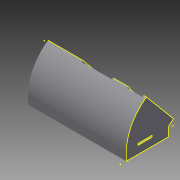
# Autodesk Inventor part: rrd display
Saved by Autodesk Inventor 2014 (Build 180170000, 170)
## iProperties
Created: 2013-09-12
Part Number: rrd display
Material: Generic
Document SubType Name: Modeling
Designer: stephen
Density: 1 g/cm^3
Appearance: Default
Author: stephen
Autodesk Inventor part; units mm, degrees
ref_plane "YZ Plane" through (0, 0, 0) normal (1, 0, 0) x (0, 1, 0)
ref_plane "XZ Plane" through (0, 0, 0) normal (0, 1, 0) x (-1, 0, 0)
ref_plane "XY Plane" through (0, 0, 0) normal (0, 0, 1) x (1, 0, 0)
sketch "Sketch1" plane through (0, 0, 0) normal (0, 0, 1) x (1, 0, 0)
  line L0 (203.8319, 85.6077) -> (27.8319, 85.6077)
  line L1 (27.8319, 85.6077) -> (27.8319, 10.1077)
  line L2 (27.8319, 10.1077) -> (203.8319, 10.1077)
  line L3 (203.8319, 10.1077) -> (203.8319, 85.6077)
  line L4 (88.1319, 64.3077) -> (185.5319, 64.3077)
  line L5 (185.5319, 64.3077) -> (185.5319, 23.9077)
  line L6 (185.5319, 23.9077) -> (88.1319, 23.9077)
  line L7 (88.1319, 23.9077) -> (88.1319, 64.3077)
  circle A0 centre (63.3719, 47.7577) radius 3.5
  circle A1 centre (63.3719, 67.0777) radius 1
  circle A2 centre (59.5619, 67.0777) radius 1
  circle A3 centre (67.1819, 67.0777) radius 1
  line L8 (65.9589, 30.9177) -> (60.7989, 30.9177) construction
  line L9 (65.9589, 33.8177) -> (60.7989, 33.8177)
  line L10 (60.7989, 28.0177) -> (65.9589, 28.0177)
  arc A4 (65.9589, 28.0177) -> (65.9589, 33.8177) centre (65.9589, 30.9177) ccw
  arc A5 (60.7989, 33.8177) -> (60.7989, 28.0177) centre (60.7989, 30.9177) ccw
  line L11 (60.7989, 30.9177) -> (65.9589, 30.9177) construction
  line L12 (60.7989, 36.3177) -> (65.9589, 36.3177)
  line L13 (65.9589, 25.5177) -> (60.7989, 25.5177)
  circle A6 centre (55.7989, 30.9177) radius 0.8
  arc A7 (55.7989, 33.8477) -> (55.7989, 27.9877) centre (55.7989, 30.9177) ccw
  line L14 (52.8689, 30.9177) -> (52.156, 30.9177)
  circle A8 centre (70.9589, 30.9177) radius 0.8
  arc A9 (70.9589, 27.9877) -> (70.9589, 33.8477) centre (70.9589, 30.9177) ccw
  line L15 (55.7989, 33.8477) -> (56.263, 33.8477)
  line L16 (55.7989, 27.9877) -> (56.263, 27.9877)
  line L17 (70.9589, 33.8477) -> (70.4949, 33.8477)
  line L18 (70.9589, 27.9877) -> (70.4949, 27.9877)
  arc A10 (65.9589, 25.5177) -> (70.4949, 27.9877) centre (65.9589, 30.9177) ccw
  arc A11 (70.4949, 33.8477) -> (65.9589, 36.3177) centre (65.9589, 30.9177) ccw
  line L19 (63.3789, 30.9177) -> (63.6989, 30.9177)
  arc A12 (60.7989, 36.3177) -> (56.263, 33.8477) centre (60.7989, 30.9177) ccw
  arc A13 (56.263, 27.9877) -> (60.7989, 25.5177) centre (60.7989, 30.9177) ccw
  line L20 (49.2039, 75.3911) -> (49.2038, 75.3911)
  line L21 (197.3319, 23.9109) -> (197.3319, 23.9077)
  line L22 (34.8319, 58.2326) -> (47.1919, 58.2326)
  line L23 (47.1919, 58.2326) -> (47.1919, 37.3026)
  line L24 (47.1919, 37.3026) -> (34.8319, 37.3026)
  line L25 (34.8319, 37.3026) -> (34.8319, 58.2326)
  line L26 (63.3719, 47.7577) -> (63.3818, 51.2577)
  line L27 (63.3719, 47.7577) -> (59.872, 47.7675)
  circle A14 centre (52.0039, 25.4109) radius 1.5
  circle A15 centre (52.0039, 75.4645) radius 1.5
  circle A16 centre (197.004, 75.4645) radius 1.5
  circle A17 centre (197.3319, 25.4109) radius 1.5
  line L28 (63.3789, 36.3177) -> (63.386, 38.8177)
  point P0 (0, 0)
  dimension "d53" = 3
  dimension "d0" = 176
  dimension "d1" = 75.5
  dimension "d2" = 97.4
  dimension "d3" = 40.4
  dimension "d4" = 13.8
  dimension "d5" = 18.3
  dimension "d6" = 21.26
  dimension "d7" = 7
  dimension "d8" = 34.15
  dimension "d9" = 10.96
  dimension "d10" = 5.8
  dimension "d11" = 0.007
  dimension "d12" = 7.94
  dimension "d16" = 1.6
  dimension "d17" = 10.8
  dimension "d19" = 2.13
  dimension "d20" = 0
  dimension "d21" = 1.6
  dimension "d22" = 2.13
  dimension "d24" = 2
  dimension "d25" = 1.81
  dimension "d26" = 1.81
  dimension "d27" = 0
  dimension "d28" = 14.82
  dimension "d36" = 0
  dimension "d43" = 5
  dimension "d44" = 5
  dimension "d45" = 12.36
  dimension "d46" = 20.93
  dimension "d47" = 7
  dimension "d50" = 3
  dimension "d51" = 3
  dimension "d52" = 3
  dimension "d55" = 10.1432
  dimension "d56" = 10.1432
  dimension "d57" = 15.3032
  dimension "d58" = 15.3032
  dimension "d184" = 2.5
  constraints: 62 end point, 20 point on circle, 17 centre point, 15 parallel, 12 tangent, 6 coincident, 6 perpendicular, 3 horizontal, 3 midpoint, 2 collinear, 2 equal radius, 2 point on line, 1 vertical alignment, 2 other
  measures "d0" distance of L0.start L0.end
  measures "d1" distance of L0.end L1.end
  measures "d2" distance of L4.start L4.end
  measures "d3" distance of L6.end L4.start
  measures "d4" distance between parallel lines of L2 L6
  measures "d5" distance between parallel lines of L3 L5
  measures "d6" distance edge to line of A0 L7
  measures "d7" diameter of A0
  measures "d8" distance edge to line of A0 L2
  measures "d10" distance between parallel lines of L9 L10
  measures "d11" horizontal distance of point (63.379, 30.918) L26.start
  measures "d12" distance edge to line of A0 L12
  measures "d16" diameter of A6
  measures "d17" distance between parallel lines of L12 L13
  measures "d19" radial gap between concentric circles of A7 A6
  measures "d20" distance from line of L14 A6.centre
  measures "d21" diameter of A8
  measures "d22" radial gap between concentric circles of A9 A8
  measures "d24" diameter of A1
  measures "d27" horizontal distance of L26.start A1.centre
  measures "d36" horizontal distance of point (52.004, 25.411) point (52.004, 75.465)
  measures "d43" distance of L8.start A8.centre
  measures "d44" distance of L8.end A6.centre
  measures "d45" distance of L22.end L22.start
  measures "d46" distance of L24.end L22.start
  measures "d47" distance from line of L1 L22.start
  measures "d50" diameter of A14
  measures "d51" diameter of A15
  measures "d52" diameter of A16
  measures "d55" distance from line of L0 point (52.004, 75.465)
  measures "d56" distance from line of L0 A16.centre
  measures "d57" distance from line of L2 point (197.332, 25.411)
  measures "d58" distance from line of L2 point (52.004, 25.411)
  measures "d184" distance of L28.start L28.end
extrude "Extrusion3" add sketch "Sketch1" along normal blind 2 contours L3 L2 L1 L0
sketch "Sketch3" plane through (0, 0, 2) normal (0, 0, 1) x (1, 0, 0)
  line L0 (203.8319, 85.6077) -> (27.8319, 85.6077) projected
  line L1 (27.8319, 85.6077) -> (27.8319, 10.1077) projected
  line L2 (27.8319, 10.1077) -> (203.8319, 10.1077) projected
  line L3 (203.8319, 10.1077) -> (203.8319, 85.6077) projected
  line L4 (30.8319, 82.6077) -> (200.8319, 82.6077)
  line L5 (200.8319, 82.6077) -> (200.8319, 13.1077)
  line L6 (200.8319, 13.1077) -> (30.8319, 13.1077)
  line L7 (30.8319, 13.1077) -> (30.8319, 82.6077)
  point P0 (0, 0)
  dimension "d63" = 3
  dimension "d64" = 3
  dimension "d65" = 3
  dimension "d66" = 3
  constraints: 8 end point, 2 parallel, 1 horizontal, 1 perpendicular
  measures "d63" distance between parallel lines of L0 L4
  measures "d64" distance between parallel lines of L2 L6
  measures "d65" distance between parallel lines of L1 L7
  measures "d66" distance between parallel lines of L3 L5
extrude "Extrusion4" add sketch "Sketch3" along normal blind 14
sketch "Sketch4" plane through (0, 0, 2) normal (0, 0, 1) x (1, 0, 0)
  circle A0 centre (52.0039, 25.4109) radius 1.5 projected
  circle A1 centre (52.0039, 75.4645) radius 1.5 projected
  circle A2 centre (197.004, 75.4645) radius 1.5 projected
  circle A3 centre (197.3319, 25.4109) radius 1.5 projected
  circle A4 centre (52.0039, 75.4645) radius 2.5
  circle A5 centre (197.004, 75.4645) radius 2.5
  circle A6 centre (197.3319, 25.4109) radius 2.5
  circle A7 centre (52.0039, 25.4109) radius 2.5
  point P0 (0, 0)
  dimension "d69" = 5
  dimension "d70" = 5
  dimension "d71" = 5
  dimension "d72" = 5
  constraints: 4 centre point, 4 coincident
  measures "d69" diameter of A4
  measures "d70" diameter of A5
  measures "d71" diameter of A6
  measures "d72" diameter of A7
sketch "Sketch5" plane through (0, 0, 0) normal (0, 0, -1) x (-1, 0, 0)
  arc A0 (-65.9589, 36.3177) -> (-70.4949, 33.8477) centre (-65.9589, 30.9177) ccw projected
  line L0 (-65.9589, 36.3177) -> (-60.7989, 36.3177) projected
  arc A1 (-56.263, 33.8477) -> (-60.7989, 36.3177) centre (-60.7989, 30.9177) ccw projected
  line L1 (-56.263, 33.8477) -> (-55.7989, 33.8477) projected
  arc A2 (-55.7989, 27.9877) -> (-55.7989, 33.8477) centre (-55.7989, 30.9177) ccw projected
  line L2 (-55.7989, 27.9877) -> (-56.263, 27.9877) projected
  arc A3 (-60.7989, 25.5177) -> (-56.263, 27.9877) centre (-60.7989, 30.9177) ccw projected
  line L3 (-60.7989, 25.5177) -> (-65.9589, 25.5177) projected
  arc A4 (-70.4949, 27.9877) -> (-65.9589, 25.5177) centre (-65.9589, 30.9177) ccw projected
  line L4 (-70.4949, 27.9877) -> (-70.9589, 27.9877) projected
  arc A5 (-70.9589, 33.8477) -> (-70.9589, 27.9877) centre (-70.9589, 30.9177) ccw projected
  line L5 (-70.9589, 33.8477) -> (-70.4949, 33.8477) projected
  point P0 (0, 0)
extrude "Extrusion5" add sketch "Sketch5" against normal blind 6.8
sketch "Sketch6" plane through (0, 0, 6.8) normal (0, 0, 1) x (1, 0, 0)
  arc A0 (55.7989, 33.8477) -> (55.7989, 27.9877) centre (55.7989, 30.9177) ccw projected
  arc A1 (70.9589, 27.9877) -> (70.9589, 33.8477) centre (70.9589, 30.9177) ccw projected
  circle A2 centre (55.7989, 30.9177) radius 0.8
  circle A3 centre (70.9589, 30.9177) radius 0.8
  point P0 (0, 0)
  dimension "d75" = 1.6
  dimension "d76" = 1.6
  constraints: 2 centre point, 2 coincident
  measures "d75" diameter of A2
  measures "d76" diameter of A3
extrude "Extrusion6" cut sketch "Sketch6" against normal blind 4.8 contours A3
sketch "Sketch7" plane through (0, 0, 6.8) normal (0, 0, 1) x (1, 0, 0)
  arc A0 (55.7989, 33.8477) -> (55.7989, 27.9877) centre (55.7989, 30.9177) ccw projected
  circle A1 centre (55.7989, 30.9177) radius 0.8
  point P0 (0, 0)
  dimension "d79" = 1.6
  constraints: 1 centre point, 1 coincident
  measures "d79" diameter of A1
extrude "Extrusion7" cut sketch "Sketch7" against normal blind 4.8
sketch "Sketch9" plane through (0, 0, 6.8) normal (0, 0, 1) x (1, 0, 0)
  line L0 (65.9589, 36.3177) -> (60.7989, 36.3177) projected
  arc A0 (56.263, 27.9877) -> (60.7989, 25.5177) centre (60.7989, 30.9177) ccw projected
  arc A1 (65.9589, 25.5177) -> (70.4949, 27.9877) centre (65.9589, 30.9177) ccw projected
  line L1 (65.9589, 30.9177) -> (60.7989, 30.9177) construction
  line L2 (65.9589, 33.8177) -> (60.7989, 33.8177)
  line L3 (60.7989, 28.0177) -> (65.9589, 28.0177)
  arc A2 (65.9589, 28.0177) -> (65.9589, 33.8177) centre (65.9589, 30.9177) ccw
  arc A3 (60.7989, 33.8177) -> (60.7989, 28.0177) centre (60.7989, 30.9177) ccw
  point P0 (0, 0)
  point P1 (63.3789, 30.9177)
  dimension "d83" = 5.8
  constraints: 8 end point, 4 point on circle, 4 tangent, 2 centre point, 2 parallel, 1 midpoint
  measures "d83" diameter of A3
extrude "Extrusion8" cut sketch "Sketch9" against normal blind 6.8
extrude "Extrusion9" add sketch "Sketch4" along normal blind 9.9 contours A7
sketch "Sketch10" plane through (0, 0, 2) normal (0, 0, 1) x (1, 0, 0)
  circle A0 centre (52.0039, 75.4645) radius 1.5 projected
  circle A1 centre (52.0039, 75.4645) radius 2.5
  point P0 (0, 0)
  dimension "d88" = 5
  constraints: 1 centre point, 1 coincident
  measures "d88" diameter of A1
extrude "Extrusion10" add sketch "Sketch10" along normal blind 9.9
sketch "Sketch11" plane through (0, 0, 2) normal (0, 0, 1) x (1, 0, 0)
  circle A0 centre (197.004, 75.4645) radius 1.5 projected
  circle A1 centre (197.004, 75.4645) radius 2.5
  point P0 (0, 0)
  dimension "d91" = 5
  constraints: 1 centre point, 1 coincident
  measures "d91" diameter of A1
extrude "Extrusion11" add sketch "Sketch11" along normal blind 9.9
sketch "Sketch12" plane through (0, 0, 2) normal (0, 0, 1) x (1, 0, 0)
  circle A0 centre (197.3319, 25.4109) radius 1.5 projected
  circle A1 centre (197.3319, 25.4109) radius 2.5
  point P0 (0, 0)
  dimension "d94" = 5
  constraints: 1 centre point, 1 coincident
  measures "d94" diameter of A1
extrude "Extrusion12" add sketch "Sketch12" along normal blind 9.9
sketch "Sketch13" plane through (27.8319, 10.1077, 0) normal (-1, 0, 0) x (0, 0, 1)
  line L0 (16, 75.5) -> (16, 0) projected
  line L1 (16, 75.5) -> (66.453, 33.1649)
  line L2 (16, 75.5) -> (81.8617, 75.5) construction
  line L3 (16, 75.5) -> (23.7135, 84.6925)
  line L4 (23.7135, 84.6925) -> (81.5498, 36.1621)
  line L5 (23.7135, 84.6925) -> (81.5498, 36.1621)
  arc A0 (16, 0) -> (81.5498, 36.1621) centre (12.2266, 84.331) ccw
  point P0 (0, -10.1077)
  dimension "d97" = 40
  dimension "d99" = 12
  dimension "d100" = 75.5
  constraints: 10 end point, 2 point on circle, 1 centre point, 1 equal length, 1 horizontal, 1 perpendicular
  measures "d97" angle of L1 L2
  measures "d99" distance of L0.start L3.end
  measures "d100" distance of L4.end L3.end
extrude "Extrusion13" add sketch "Sketch13" against normal blind 3
sketch "Sketch14" plane through (203.8319, 10.1077, 0) normal (1, 0, 0) x (0, 0, -1)
  line L0 (-16, 0) -> (-16, 75.5) projected
  line L1 (-16, 75.5) -> (-23.7135, 84.6925)
  line L2 (-16, 75.5) -> (-4, 75.5) construction
  line L3 (-23.7135, 84.6925) -> (-81.5498, 36.1621)
  arc A0 (-81.5498, 36.1621) -> (-16, 0) centre (-12.2268, 84.3306) ccw
  point P0 (0, -10.1077)
  dimension "d103" = 12
  dimension "d104" = 130
  dimension "d105" = 75.5
  dimension "d106" = 84.415
  constraints: 6 end point, 2 point on circle, 1 centre point, 1 equal length, 1 horizontal, 1 perpendicular
  measures "d103" distance of L0.end L1.end
  measures "d104" angle of L2 L1
  measures "d105" distance of L1.end L3.end
  measures "d106" radius of A0
extrude "Extrusion14" add sketch "Sketch14" along normal blind 3
sketch "Sketch15" plane through (30.8319, 13.1077, 2) normal (1, 0, 0) x (0, 0, -1)
  line L0 (-14, 72.5) -> (-14, 69.5) projected
  line L1 (-14, 72.5) -> (-21.7135, 81.6925) projected
  line L2 (-21.7135, 81.6925) -> (-79.5498, 33.1621) projected
  arc A0 (-79.5498, 33.1621) -> (-14, -3) centre (-10.2266, 81.331) ccw projected
  line L3 (-14, 0) -> (-14, -3) projected
  line L4 (-14, 69.5) -> (-21.2623, 78.1549)
  line L5 (-21.2623, 78.1549) -> (-75.4966, 32.6469)
  line L6 (-79.5498, 33.1621) -> (-77.2517, 35.0904)
  arc A1 (-75.4966, 32.6469) -> (-14, 0) centre (-10.203, 81.396) ccw
  point P0 (2, -13.1077)
  dimension "d110" = 3
  dimension "d111" = 3
  constraints: 6 end point, 2 perpendicular, 2 point on circle, 1 centre point, 1 point on line
  measures "d110" distance of L2.end L6.end
extrude "Extrusion15" add sketch "Sketch15" along normal blind 173
sketch "Sketch16" plane through (27.8319, 94.8002, 23.7135) normal (0, 0.7660444, 0.6427876) x (1, 0, 0)
  line L0 (179, 0) -> (179, -75.5) projected
  line L1 (0, 0) -> (179, 0) projected
  line L2 (0, -75.5) -> (0, 0) projected
  line L3 (0, -75.5) -> (176, -75.5) projected
  line L4 (3, -3) -> (176, -3)
  line L5 (176, -3) -> (176, -72.5)
  line L6 (176, -72.5) -> (3, -72.5)
  line L7 (3, -72.5) -> (3, -3)
  point P0 (-27.8319, -42.7709)
  dimension "d114" = 3
  dimension "d115" = 3
  dimension "d116" = 3
  dimension "d117" = 3
  constraints: 8 end point, 2 parallel, 1 horizontal, 1 perpendicular
  measures "d114" distance between parallel lines of L2 L7
  measures "d115" distance between parallel lines of L0 L5
  measures "d116" distance between parallel lines of L1 L4
  measures "d117" distance between parallel lines of L3 L6
extrude "Extrusion16" cut sketch "Sketch16" against normal blind 3
sketch "Sketch17" plane through (27.8319, 94.8002, 23.7135) normal (0, 0.7660444, 0.6427876) x (1, 0, 0)
  line L0 (3, -3) -> (176, -3) projected
  line L1 (47.9345, -3) -> (63.9345, -3)
  line L2 (63.9345, -3) -> (63.9345, -13.34)
  line L3 (63.9345, -13.34) -> (47.9345, -13.34)
  line L4 (47.9345, -13.34) -> (47.9345, -3)
  circle A0 centre (55.9345, -8.17) radius 2.55
  circle A1 centre (126.5095, -8.17) radius 2.55
  line L5 (126.5095, -3) -> (118.5095, -3)
  line L6 (118.5095, -3) -> (134.5095, -3)
  line L7 (134.5095, -3) -> (134.5095, -13.34)
  line L8 (134.5095, -13.34) -> (118.5095, -13.34)
  line L9 (118.5095, -13.34) -> (118.5095, -3)
  line L10 (56.4995, -3) -> (47.9345, -3)
  line L11 (134.5095, -3) -> (118.5095, -3)
  line L12 (55.9345, -13.34) -> (55.9345, -10.72)
  line L13 (176, -3) -> (176, -72.5) projected
  line L14 (0, -75.5) -> (176, -75.5) projected
  line L15 (126.5095, -13.34) -> (126.5095, -3)
  point P0 (-27.8319, -42.7709)
  dimension "d124" = 5.1
  dimension "d120" = 16
  dimension "d122" = 10.34
  dimension "d125" = 75.675
  dimension "d127" = 8
  dimension "d128" = 16
  dimension "d131" = 8.565
  dimension "d185" = 0
  dimension "d186" = 49.4905
  constraints: 26 end point, 4 parallel, 3 perpendicular, 2 horizontal, 2 midpoint, 1 centre point, 1 collinear, 1 point on line, 1 vertical alignment, 2 other
  measures "d120" distance between parallel lines of L4 L2
  measures "d122" distance of L1.end L2.end
  measures "d127" distance of L5.start L5.end
  measures "d128" distance of L7.end L8.end
  measures "d131" distance of L10.start L10.end
  measures "d185" distance from line of L15 A1.centre
  measures "d186" distance from line of A1.centre L13
extrude "Extrusion17" add sketch "Sketch17" against normal blind 3 contours L0 L15 A1 L8 L9 | L0 L7 L8 L15 A1
sketch "Sketch18" plane through (27.8319, 94.8002, 23.7135) normal (0, 0.7660444, 0.6427876) x (1, 0, 0)
  circle A0 centre (126.5095, -8.17) radius 2.55 projected
  line L0 (3, -72.5) -> (3, -3) projected
  line L1 (3, -3) -> (118.5095, -3) projected
  line L2 (44.49, -3) -> (60.49, -3)
  line L3 (60.49, -3) -> (60.49, -13.34)
  line L4 (60.49, -13.34) -> (44.49, -13.34)
  line L5 (44.49, -13.34) -> (44.49, -3)
  circle A1 centre (52.4895, -8.17) radius 2.55
  line L6 (60.49, -13.34) -> (52.49, -13.34)
  line L7 (52.49, -3) -> (52.49, -13.34)
  point P0 (-27.8319, -42.7709)
  dimension "d134" = 5.1
  dimension "d135" = 10.34
  dimension "d136" = 16
  dimension "d137" = 0
  dimension "d138" = 41.49
  dimension "d187" = 79.12
  constraints: 12 end point, 2 midpoint, 2 parallel, 2 perpendicular, 1 centre point, 1 horizontal, 1 point on line
  measures "d134" diameter of A1
  measures "d135" distance of L2.end L3.end
  measures "d136" distance of L3.end L4.end
  measures "d137" vertical distance of A1.centre A0.centre
  measures "d138" distance between parallel lines of L0 L5
extrude "Extrusion18" add sketch "Sketch18" against normal blind 3 contours L1 L7 A1 L4 L5 | L1 L3 L4 L7 A1
sketch "Sketch19" plane through (0, 0, 0) normal (0, 0, -1) x (-1, 0, 0)
  circle A0 centre (-197.004, 75.4645) radius 1.5 projected
  circle A1 centre (-197.004, 75.4645) radius 1.5
  point P0 (0, 0)
  constraints: 1 centre point, 1 coincident, 1 concentric
extrude "Extrusion19" add sketch "Sketch19" against normal blind 3
sketch "Sketch20" plane through (0, 0, 0) normal (0, 0, -1) x (-1, 0, 0)
  circle A0 centre (-197.3319, 25.4109) radius 1.5 projected
  circle A1 centre (-197.3319, 25.4109) radius 1.5
  point P0 (0, 0)
  constraints: 1 centre point, 1 coincident, 1 concentric
extrude "Extrusion20" add sketch "Sketch20" against normal blind 3
sketch "Sketch21" plane through (0, 0, 0) normal (0, 0, -1) x (-1, 0, 0)
  circle A0 centre (-52.0039, 25.4109) radius 1.5 projected
  circle A1 centre (-52.0039, 25.4109) radius 1.5
  point P0 (0, 0)
  constraints: 1 centre point, 1 coincident, 1 concentric
extrude "Extrusion21" add sketch "Sketch21" against normal blind 3
sketch "Sketch22" plane through (0, 0, 0) normal (0, 0, -1) x (-1, 0, 0)
  circle A0 centre (-52.0039, 75.4645) radius 1.5 projected
  circle A1 centre (-52.0039, 75.4645) radius 1.5
  point P0 (0, 0)
  constraints: 1 centre point, 1 coincident, 1 concentric
extrude "Extrusion22" add sketch "Sketch22" against normal blind 3
sketch "Sketch23" plane through (27.8319, 94.8002, 23.7135) normal (0, 0.7660444, 0.6427876) x (1, 0, 0)
  circle A0 centre (52.4895, -8.17) radius 2.55 projected
  line L0 (44.49, -13.34) -> (60.49, -13.34) projected
  line L1 (176, -72.5) -> (3, -72.5) projected
  line L2 (60.49, -13.34) -> (60.49, -72.5)
  line L3 (44.49, -15.3523) -> (44.49, -72.5)
  line L4 (60.49, -72.5) -> (44.49, -72.5)
  line L5 (44.49, -72.5) -> (44.49, -58.5)
  line L6 (60.49, -58.5) -> (60.49, -72.5)
  circle A1 centre (52.4895, -58.57) radius 2.55
  line L7 (44.49, -13.34) -> (44.49, -16.6172)
  point P0 (-27.8319, -42.7709)
  dimension "d151" = 5.1
  dimension "d153" = 55.5
  constraints: 12 end point, 4 point on line, 3 perpendicular, 1 centre point, 1 horizontal, 1 parallel
  measures "d151" diameter of A1
extrude "Extrusion23" add sketch "Sketch23" against normal blind 3 contours L0 L2 L1 L3 L7
sketch "Sketch24" plane through (27.8319, 94.8002, 23.7135) normal (0, 0.7660444, 0.6427876) x (1, 0, 0)
  circle A0 centre (126.5095, -8.17) radius 2.55 projected
  line L0 (118.5095, -13.34) -> (134.5095, -13.34) projected
  line L1 (176, -72.5) -> (60.49, -72.5) projected
  line L2 (134.5095, -13.34) -> (134.5095, -72.5)
  line L3 (118.5095, -13.34) -> (118.5095, -72.5)
  circle A1 centre (126.5095, -58.57) radius 2.55
  point P0 (-27.8319, -42.7709)
  dimension "d156" = 55.5
  dimension "d157" = 5.1
  constraints: 4 end point, 2 perpendicular, 2 point on line, 1 centre point
  measures "d157" diameter of A1
extrude "Extrusion24" add sketch "Sketch24" against normal blind 3 contours L0 L2 L1 L3
sketch "Sketch25" plane through (203.8319, 10.1077, 0) normal (-1, 0, 0) x (0, 0, 1)
  line L0 (23.2623, 81.1549) -> (16, 72.5) projected
  line L1 (16, 3) -> (16, 72.5) projected
  arc A0 (16, 3) -> (77.4966, 35.6469) centre (12.203, 84.396) ccw projected
  line L2 (77.4966, 35.6469) -> (77.3233, 35.7923) projected
  line L3 (79.2517, 38.0904) -> (77.3233, 35.7923) projected
  line L4 (26.0116, 82.7642) -> (79.2517, 38.0904) projected
  line L5 (26.0116, 82.7642) -> (24.0832, 80.466) projected
  line L6 (24.0832, 80.466) -> (23.2623, 81.1549) projected
  point P0 (0, -10.1077)
extrude "Extrusion25" add sketch "Sketch25" along normal blind 3
sketch "Sketch26" plane through (206.8319, 10.1077, 0) normal (1, 0, 0) x (0, 0, -1)
  line L0 (-16, 75.5) -> (-23.7135, 84.6925) projected
  line L1 (-23.7135, 84.6925) -> (-81.5498, 36.1621) projected
  arc A0 (-81.5498, 36.1621) -> (-16, 0) centre (-12.2268, 84.3306) ccw projected
  line L2 (-16, 0) -> (-16, 75.5) projected
  point P0 (0, -10.1077)
extrude "Extrusion26" cut sketch "Sketch26" against normal blind 3
sketch "Sketch27" plane through (203.8319, 10.1077, 0) normal (1, 0, 0) x (0, 0, -1)
  line L0 (0, 0) -> (0, 75.5) projected
  line L1 (0, 0) -> (0, 21.2)
  line L2 (0, 21.2) -> (0, 46.2)
  line L3 (0, 21.2) -> (-14.2, 21.2)
  line L4 (-14.2, 21.2) -> (-17.1, 21.2)
  line L5 (-17.1, 21.2) -> (-17.1, 46.2)
  line L6 (-17.1, 46.2) -> (-14.2, 46.2)
  line L7 (-14.2, 46.2) -> (-14.2, 21.2)
  point P0 (0, -10.1077)
  dimension "d164" = 21.2
  dimension "d165" = 25
  dimension "d166" = 14.2
  dimension "d167" = 2.9
  constraints: 14 end point, 2 parallel, 2 perpendicular, 2 point on line, 1 horizontal
  measures "d164" distance of L0.start L1.end
  measures "d165" distance of L1.end L2.end
  measures "d166" distance of L1.end L3.end
  measures "d167" distance of L5.end L6.end
extrude "Extrusion27" cut sketch "Sketch27" against normal blind 3
sketch "Sketch28" plane through (200.8319, 48.1981, 79.2517) normal (0, 0.6427876, -0.7660444) x (-1, 0, 0)
  line L0 (0, 0) -> (38.4905, 0) projected
  line L1 (0, 0) -> (2, 0)
  line L2 (2, 0) -> (29, 0)
  line L3 (29, 0) -> (29, -2.5)
  line L4 (29, -2.5) -> (2, -2.5)
  line L5 (2, -2.5) -> (2, 0)
  point P0 (200.8319, -87.8639)
  dimension "d170" = 2
  dimension "d171" = 27
  dimension "d172" = 2.5
  constraints: 10 end point, 2 parallel, 1 horizontal, 1 perpendicular, 1 point on line
  measures "d170" distance of L0.start L1.end
  measures "d171" distance of L3.end L4.end
  measures "d172" distance of L2.end L3.end
extrude "Extrusion28" cut sketch "Sketch28" against normal blind 3.1
sketch "Sketch29" plane through (146.3414, 48.1981, 79.2517) normal (0, 0.6427876, -0.7660444) x (-1, 0, 0)
  line L0 (58.0195, -3) -> (0, -3) projected
  line L1 (0, 0) -> (58.0195, 0) projected
  line L2 (0, 0) -> (2, 0)
  line L3 (58.0195, 0) -> (56.0195, 0)
  line L4 (2, 0) -> (56.0195, 0)
  line L5 (56.0195, 0) -> (56.0195, -2.5)
  line L6 (56.0195, -2.5) -> (2, -2.5)
  line L7 (2, -2.5) -> (2, 0)
  point P0 (146.3414, -87.8639)
  dimension "d175" = 2
  dimension "d176" = 2
  dimension "d177" = 2.5
  constraints: 12 end point, 3 parallel, 2 point on line, 1 perpendicular
  measures "d175" distance of L1.start L2.end
  measures "d176" distance of L1.end L3.end
  measures "d177" distance of L3.end L5.end
extrude "Extrusion29" cut sketch "Sketch29" against normal blind 3
sketch "Sketch30" plane through (146.3414, 46.2698, 81.5498) normal (0, 0.6427876, -0.7660444) x (-1, 0, 0)
  line L0 (2, -2.5) -> (2, 0) projected
  line L1 (56.0195, -2.5) -> (2, -2.5) projected
  line L2 (56.0195, 0) -> (56.0195, -2.5) projected
  line L3 (56.0195, 0) -> (2, 0) projected
  line L4 (2, 0) -> (56.0195, 0)
  line L5 (56.0195, 0) -> (56.0195, -2.5)
  line L6 (56.0195, -2.5) -> (2, -2.5)
  line L7 (2, -2.5) -> (2, 0)
  point P0 (146.3414, -87.8639)
  constraints: 8 end point, 3 equal length, 1 perpendicular
extrude "Extrusion30" cut sketch "Sketch30" against normal blind 0.25
sketch "Sketch31" plane through (200.8319, 46.2055, 81.6264) normal (0, 0.6427876, -0.7660444) x (-1, 0, 0)
  line L0 (2, -1.1906) -> (29, -1.1906) projected
  line L1 (2, -1.1906) -> (29, -1.1906)
  line L2 (29, -1.1906) -> (29, -2.5)
  line L3 (29, -2.5) -> (2, -2.5)
  line L4 (2, -2.5) -> (2, -1.1906)
  point P0 (200.8319, -87.8639)
  constraints: 8 end point, 3 equal length, 1 perpendicular
extrude "Extrusion31" cut sketch "Sketch31" against normal blind 0.25
sketch "Sketch33" plane through (203.8319, 10.1077, 0) normal (1, 0, 0) x (0, 0, -1)
  line L0 (-17.1, 46.2) -> (-14.2, 46.2) projected
  line L1 (-14.2, 46.2) -> (-14.2, 21.2) projected
  line L2 (-14.2, 21.2) -> (-17.1, 21.2) projected
  line L3 (-17.1, 21.2) -> (-17.1, 46.2) projected
  line L4 (0, 0) -> (0, 75.5) projected
  line L5 (0, 75.5) -> (-16, 75.5) projected
  line L6 (-23.7135, 84.6925) -> (-16, 75.5) projected
  line L7 (-81.5498, 36.1621) -> (-23.7135, 84.6925) projected
  arc A0 (-81.5498, 36.1621) -> (-16, 0) centre (-12.2266, 84.331) ccw projected
  line L8 (0, 0) -> (-16, 0) projected
  point P0 (0, -10.1077)
sketch "Sketch34" plane through (27.8319, 94.8002, 23.7135) normal (0, 0.7660444, 0.6427876) x (1, 0, 0)
  circle A0 centre (126.5095, -58.57) radius 2.55 projected
  line L0 (44.49, -72.5) -> (3, -72.5) projected
  line L1 (3, -72.5) -> (3, -3) projected
  line L2 (3, -3) -> (44.49, -3) projected
  line L3 (44.49, -3) -> (44.49, -72.5) projected
  circle A1 centre (52.4895, -58.57) radius 2.55 projected
  circle A2 centre (52.4895, -8.17) radius 2.55 projected
  circle A3 centre (126.5095, -8.17) radius 2.55 projected
  line L4 (116.5095, -72.5) -> (116.5095, -75.5) projected
  line L5 (116.5095, -75.5) -> (144, -75.5) projected
  line L6 (144, -75.5) -> (144, -72.5) projected
  line L7 (144, -72.5) -> (134.5095, -72.5) projected
  line L8 (134.5095, -72.5) -> (134.5095, -3) projected
  line L9 (134.5095, -3) -> (173, -3) projected
  line L10 (173, -72.5) -> (173, -3) projected
  line L11 (173, -72.5) -> (171, -72.5) projected
  line L12 (171, -72.5) -> (171, -75.5) projected
  line L13 (171, -75.5) -> (176, -75.5) projected
  line L14 (176, -75.5) -> (176, 0) projected
  line L15 (0, 0) -> (176, 0) projected
  line L16 (0, -75.5) -> (0, 0) projected
  line L17 (0, -75.5) -> (62.49, -75.5) projected
  line L18 (62.49, -75.5) -> (62.49, -72.5) projected
  line L19 (62.49, -72.5) -> (60.49, -72.5) projected
  line L20 (60.49, -72.5) -> (60.49, -3) projected
  line L21 (60.49, -3) -> (118.5095, -3) projected
  line L22 (118.5095, -3) -> (118.5095, -72.5) projected
  line L23 (118.5095, -72.5) -> (116.5095, -72.5) projected
  point P0 (-27.8319, -42.7709)
body "Solid3"
